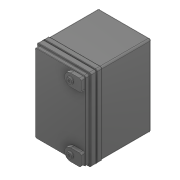
# Autodesk Inventor part: accu
Saved by Autodesk Inventor 2020.3 (Build 243373000, 373)
## iProperties
Created: 2020-09-18
Part Number: accu
Material: ABS Plastic
Document SubType Name: Modeling
Designer: Svend
Density: 1.06 g/cm^3
Appearance: Smooth - White
Author: Svend
Autodesk Inventor part; units mm, degrees
ref_plane "YZ Plane" through (0, 0, 0) normal (1, 0, 0) x (0, 1, 0)
ref_plane "XZ Plane" through (0, 0, 0) normal (0, 1, 0) x (-1, 0, 0)
ref_plane "XY Plane" through (0, 0, 0) normal (0, 0, 1) x (1, 0, 0)
sketch "Sketch1" plane through (0, 0, 0) normal (0, 0, 1) x (1, 0, 0)
  line L0 (-63.5, 97) -> (63.5, 97)
  line L1 (63.5, 97) -> (63.5, -97)
  line L2 (63.5, -97) -> (-63.5, -97)
  line L3 (-63.5, -97) -> (-63.5, 97)
  line L4 (-63.5, 97) -> (63.5, -97) construction
  line L5 (63.5, 97) -> (-63.5, -97) construction
  point P0 (0, 0)
  dimension "d0" = 127
  dimension "d1" = 194
  constraints: 12 end point, 2 midpoint, 2 parallel, 1 horizontal, 1 perpendicular
  measures "d0" distance of L1.end L2.end
  measures "d1" distance of L0.end L1.end
extrude "Extrusion1" add sketch "Sketch1" along normal blind 120
sketch "Sketch2" plane through (0, 0, 120) normal (0, 0, 1) x (1, 0, 0)
  line L0 (-63.5, -97) -> (63.5, -97) projected
  line L1 (63.5, -97) -> (63.5, 97) projected
  line L2 (63.5, 97) -> (-63.5, 97) projected
  line L3 (-63.5, 97) -> (-63.5, -97) projected
  line L4 (-64.5, -98) -> (64.5, -98)
  line L5 (64.5, -98) -> (64.5, 98)
  line L6 (64.5, 98) -> (-64.5, 98)
  line L7 (-64.5, 98) -> (-64.5, -98)
  point P0 (0, 0)
  dimension "d4" = 1
  constraints: 8 end point, 3 other
  measures "d4" distance between parallel lines of L3 L7
extrude "Extrusion2" add sketch "Sketch2" along normal blind 12 contours L3 L2 L1 L0 | L7 L6 L5 L4
sketch "Sketch3" plane through (0, 0, 132) normal (0, 0, 1) x (1, 0, 0)
  line L0 (64.5, -98) -> (64.5, 98) projected
  line L1 (64.5, 98) -> (-64.5, 98) projected
  line L2 (-64.5, 98) -> (-64.5, -98) projected
  line L3 (-64.5, -98) -> (64.5, -98) projected
  line L4 (-59.5, -93) -> (-59.5, 93)
  line L5 (-59.5, 93) -> (59.5, 93)
  line L6 (59.5, 93) -> (59.5, -93)
  line L7 (59.5, -93) -> (-59.5, -93)
  point P0 (0, 0)
  dimension "d7" = 5
  constraints: 8 end point, 3 other
  measures "d7" distance between parallel lines of L2 L4
extrude "Extrusion3" add sketch "Sketch3" along normal blind 2.5 contours L4 L5 L6 L7
sketch "Sketch4" plane through (0, 0, 134.5) normal (0, 0, 1) x (1, 0, 0)
  line L0 (59.5, -93) -> (-59.5, -93) projected
  line L1 (-59.5, -93) -> (-59.5, 93) projected
  line L2 (-59.5, 93) -> (59.5, 93) projected
  line L3 (59.5, 93) -> (59.5, -93) projected
  line L4 (64.5, -98) -> (64.5, 98) projected
  line L5 (64.5, 98) -> (-64.5, 98) projected
  line L6 (-64.5, 98) -> (-64.5, -98) projected
  line L7 (-64.5, -98) -> (64.5, -98) projected
  point P0 (0, 0)
extrude "Extrusion4" add sketch "Sketch4" along normal blind 12 contours L0 L1 L2 L3 | L7 L6 L5 L4
sketch "Sketch5" plane through (0, 0, 146.5) normal (0, 0, 1) x (1, 0, 0)
  line L0 (64.5, 98) -> (-64.5, 98) projected
  line L1 (-64.5, 98) -> (-64.5, -98) projected
  line L2 (-64.5, -98) -> (64.5, -98) projected
  line L3 (64.5, -98) -> (64.5, 98) projected
  line L4 (-60.5, 94) -> (60.5, 94)
  line L5 (60.5, 94) -> (60.5, -94)
  line L6 (60.5, -94) -> (-60.5, -94)
  line L7 (-60.5, -94) -> (-60.5, 94)
  point P0 (0, 0)
  dimension "d12" = 4
  constraints: 8 end point, 3 other
  measures "d12" distance between parallel lines of L0 L4
extrude "Extrusion5" add sketch "Sketch5" along normal blind 8.5 contours L4 L5 L6 L7
sketch "Sketch6" plane through (0, 0, 155) normal (0, 0, 1) x (1, 0, 0)
  line L0 (-60.5, -94) -> (60.5, -94) projected
  line L1 (60.5, -94) -> (60.5, 94) projected
  line L2 (60.5, 94) -> (-60.5, 94) projected
  line L3 (-60.5, 94) -> (-60.5, -94) projected
  line L4 (58.5, -92) -> (33.5, -92)
  line L5 (33.5, -92) -> (33.5, -63)
  line L6 (33.5, -63) -> (58.5, -63)
  line L7 (58.5, -63) -> (58.5, -92)
  circle A0 centre (33.5, -77.5) radius 14.5
  line L8 (-60.5, 94) -> (-60.5, -94) construction
  line L9 (-60.5, 0) -> (60.5, 0) construction
  line L10 (60.5, -94) -> (60.5, 94) construction
  line L11 (58.5, 92) -> (33.5, 92)
  line L12 (33.5, 92) -> (33.5, 63)
  line L13 (33.5, 63) -> (58.5, 63)
  line L14 (58.5, 63) -> (58.5, 92)
  circle A1 centre (33.5, 77.5) radius 14.5
  point P0 (0, 0)
  dimension "d15" = 29
  dimension "d16" = 2
  dimension "d17" = 2
  dimension "d18" = 25
  constraints: 18 end point, 5 symmetric about line, 3 midpoint, 2 horizontal, 2 parallel, 1 perpendicular, 6 other
  measures "d15" distance between parallel lines of L4 L6
  measures "d16" distance between parallel lines of L1 L7
  measures "d17" distance between parallel lines of L0 L4
  measures "d18" distance of L5.end L6.end
extrude "Extrusion6" add sketch "Sketch6" along normal blind 8.8 contours L4 A0 L6 L7 | A0 L5 | L5 A0 | L14 L13 A1 L11 | A1 L12 | L12 A1
sketch "Sketch7" plane through (0, 0, 163.8) normal (0, 0, 1) x (1, 0, 0)
  line L0 (33.5, 63) -> (58.5, 63) projected
  line L1 (58.5, 63) -> (58.5, 92) projected
  line L2 (58.5, 92) -> (33.5, 92) projected
  arc A0 (33.5, 92) -> (33.5, 63) centre (33.5, 77.5) ccw projected
  line L3 (33.5, -92) -> (58.5, -92) projected
  line L4 (58.5, -92) -> (58.5, -63) projected
  line L5 (58.5, -63) -> (33.5, -63) projected
  arc A1 (33.5, -63) -> (33.5, -92) centre (33.5, -77.5) ccw projected
  circle A2 centre (33.5, -77.5) radius 7
  circle A3 centre (33.5, 77.5) radius 7
  point P0 (0, 0)
  dimension "d21" = 14
  dimension "d22" = 14
  constraints: 2 centre point, 2 coincident
  measures "d21" diameter of A2
  measures "d22" diameter of A3
extrude "Extrusion7" add sketch "Sketch7" along normal blind 4 contours A2 | A3
sketch "Sketch8" plane through (33.5, 77.5, 167.8) normal (0, 0, 1) x (1, 0, 0)
  circle A0 centre (0, 0) radius 7 projected
  circle A1 centre (0, -155) radius 7 projected
  point P0 (-33.5, -77.5)
  constraints: 2 coincident
hole "Hole1" at (33.5, 77.5, 167.8) at (33.5, -77.5, 167.8) direction (0, 0, -1) diameter 4.917 depth 17.1 tip angle 90 thread size "M6x1" class "6H" standard "ISO Metric profile"
fillet "Fillet1" radius 4 4 edges at (63.5, -97, 60) (63.5, 97, 60) (-63.5, -97, 60) (-63.5, 97, 60)
fillet "Fillet2" radius 4 8 edges at (-62.3284, -95.8284, 0) (0, -97, 0) (62.3284, -95.8284, 0) (63.5, 0, 0) (62.3284, 95.8284, 0) (0, 97, 0) (-62.3284, 95.8284, 0) (-63.5, 0, 0)
fillet "Fillet3" radius 4 16 edges at (-64.5, 98, 126) (-64.5, 98, 140.5) (64.5, 98, 126) (64.5, 98, 140.5) (64.5, -98, 126) (64.5, -98, 140.5) (-64.5, -98, 126) (-64.5, -98, 140.5) (-60.5, -94, 150.75) (60.5, -94, 150.75) (58.5, -92, 159.4) (58.5, -63, 159.4) (58.5, 63, 159.4) (58.5, 92, 159.4) (60.5, 94, 150.75) (-60.5, 94, 150.75)
fillet "Fillet4" radius 1 48 edges at (-59.3284, -92.8284, 155) (0, -94, 155) (59.3284, -92.8284, 155) (60.5, 0, 155) (59.3284, 92.8284, 155) (0, 94, 155) (-59.3284, 92.8284, 155) (-60.5, 0, 155) (-59.3284, 92.8284, 146.5) (0, 94, 146.5) (59.3284, 92.8284, 146.5) (60.5, 0, 146.5) (59.3284, -92.8284, 146.5) (0, -94, 146.5) (-59.3284, -92.8284, 146.5) (-60.5, 0, 146.5) (-63.3284, -96.8284, 146.5) (0, -98, 146.5) (63.3284, -96.8284, 146.5) (64.5, 0, 146.5) (63.3284, 96.8284, 146.5) (0, 98, 146.5) (-63.3284, 96.8284, 146.5) (-64.5, 0, 146.5) (-63.3284, -96.8284, 132) (0, -98, 132) (63.3284, -96.8284, 132) (64.5, 0, 132) (63.3284, 96.8284, 132) (0, 98, 132) (-63.3284, 96.8284, 132) (-64.5, 0, 132) (-63.3284, -96.8284, 120) (0, -98, 120) (63.3284, -96.8284, 120) (64.5, 0, 120) (63.3284, 96.8284, 120) (0, 98, 120) (-63.3284, 96.8284, 120) (-64.5, 0, 120) (-62.3284, 95.8284, 120) (-63.5, 0, 120) (-62.3284, -95.8284, 120) (0, -97, 120) (62.3284, -95.8284, 120) (63.5, 0, 120) (62.3284, 95.8284, 120) (0, 97, 120)
fillet "Fillet5" radius 1 2 edges at (26.5, 77.5, 163.8) (26.5, -77.5, 163.8)
equation "\"d17\" = d16"
body "Solid1"
